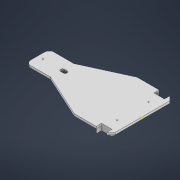
# Autodesk Inventor part: Base
Saved by Autodesk Inventor 2022 (Build 260153000, 153)
## iProperties
Created: 2022-06-09
Part Number: Base
Material: Generic
Document SubType Name: Modeling
Designer: Gugarauj07
Density: 1 g/cm^3
Appearance: Default
Author: Gugarauj07
Autodesk Inventor part; units mm, degrees
ref_plane "YZ Plane" through (0, 0, 0) normal (1, 0, 0) x (0, 1, 0)
ref_plane "XZ Plane" through (0, 0, 0) normal (0, 1, 0) x (-1, 0, 0)
ref_plane "XY Plane" through (0, 0, 0) normal (0, 0, 1) x (1, 0, 0)
sketch "Sketch1" plane through (0, 0, 0) normal (0, 1, 0) x (-1, 0, 0)
  line L0 (0, 0) -> (0, 300)
  line L1 (0, 300) -> (350, 300)
  line L2 (350, 300) -> (1000, 100)
  line L3 (0, 0) -> (1000, 0)
  line L4 (1000, 100) -> (1000, 0)
  line L5 (0, 0) -> (0, -300)
  line L6 (0, -300) -> (350, -300)
  line L7 (350, -300) -> (1000, -100)
  line L8 (1000, -100) -> (1000, 0)
  line L9 (350, 300) -> (350, -300)
  dimension "d12" = 300
  dimension "d13" = 350
  dimension "d16" = 100
  constraints: 20 end point, 3 symmetric about line, 2 vertical, 1 horizontal, 1 perpendicular
  measures "d12" distance of L0.start L0.end
  measures "d13" distance of L0.end L1.end
  measures "d16" distance of L2.end L3.end
extrude "Extrusion1" add sketch "Sketch1" along normal blind 20
fillet "Fillet1" radius 50 1 edges at (-1000, 10, 100)
fillet "Fillet2" radius 50 1 edges at (-1000, 10, -100)
chamfer "Chamfer1" distance 40 angle 45 1 edges at (0, 10, -300)
chamfer "Chamfer2" distance 40 angle 45 1 edges at (0, 10, 300)
sketch "Sketch3" plane through (0, 20, 0) normal (0, 1, 0) x (1, 0, 0)
  point P0 (0, 0)
sketch "Sketch4" plane through (0, 20, 0) normal (0, 1, 0) x (1, 0, 0)
  point P0 (0, 0)
sketch "Sketch5" plane through (0, 20, 0) normal (0, 1, 0) x (1, 0, 0)
  line L0 (-780, 0) -> (-720, 0) construction
  line L1 (-762.5, -17.5) -> (-737.5, -17.5)
  line L2 (-737.5, 17.5) -> (-762.5, 17.5)
  arc A0 (-762.5, 17.5) -> (-762.5, -17.5) centre (-762.5, 0) ccw
  arc A1 (-737.5, -17.5) -> (-737.5, 17.5) centre (-737.5, 0) ccw
  line L3 (-1000, 63.0713) -> (-1000, -63.0713) projected
  point P0 (0, 0)
  point P1 (-750, 0)
  dimension "d27" = 60
  dimension "d28" = 35
  constraints: 8 end point, 6 point on circle, 4 tangent, 2 centre point, 2 point on line, 1 horizontal, 1 midpoint, 1 parallel
  measures "d27" distance of L0.start L0.end
  measures "d28" diameter of A1
extrude "Extrusion2" cut sketch "Sketch5" against normal blind 20
sketch "Sketch6" plane through (0, 20, 0) normal (0, 1, 0) x (1, 0, 0)
  line L0 (-1000, 63.0713) -> (-1000, -63.0713) projected
  line L1 (-1000, 0) -> (-950, 0)
  point P0 (0, 0)
  dimension "d33" = 50
  constraints: 2 end point, 1 horizontal, 1 midpoint
  measures "d33" distance of L1.start L1.end
hole "Hole1" at (-950, 20, 0) direction (0, -1, 0) diameter 10 end through all
sketch "Sketch7" plane through (0, 0, 0) normal (0, -1, 0) x (1, 0, 0)
  line L0 (-350, 300) -> (-40, 300) projected
  line L1 (0, -260) -> (-40, -300) projected
  line L2 (-40, 300) -> (-40, -300)
  line L3 (-40, -300) -> (-140, -300)
  line L4 (-140, -300) -> (-140, 300)
  line L5 (-140, 300) -> (-40, 300)
  point P0 (0, 0)
  dimension "d41" = 100
  constraints: 8 end point, 2 parallel, 1 perpendicular, 1 vertical
  measures "d41" distance of L1.end L3.end
extrude "Extrusion3" add sketch "Sketch7" along normal blind 40
sketch "Sketch8" plane through (0, -40, 0) normal (0, -1, 0) x (1, 0, 0)
  line L0 (-350, 300) -> (-40, 300) projected
  circle A0 centre (-91.5513, 150) radius 5
  line L1 (-40, -300) -> (-40, 300) projected
  line L2 (-40, 0) -> (-140, 0)
  line L3 (-140, -300) -> (-140, 300) projected
  circle A1 centre (-91.5513, -150) radius 5
  point P0 (0, 0)
  dimension "d45" = 10
  constraints: 2 centre point, 2 end point, 2 midpoint, 1 symmetric about line, 1 other
  measures "d45" diameter of A0
extrude "Extrusion4" cut sketch "Sketch8" against normal blind 60 contours A0 | A1
sketch "Sketch9" plane through (0, -40, 0) normal (0, -1, 0) x (1, 0, 0)
  line L0 (-40, -300) -> (-350, -300) projected
  line L1 (-139.5196, -300) -> (-39.5196, -300)
  line L2 (-39.5196, -300) -> (-39.5196, -250)
  line L3 (-39.5196, -250) -> (-139.5196, -250)
  line L4 (-139.5196, -250) -> (-139.5196, -300)
  line L5 (-40, -300) -> (-40, 300) projected
  line L6 (-40, 0) -> (-139.5196, 0)
  line L7 (-40, 300) -> (-350, 300)
  line L8 (-39.5196, 300) -> (-39.5196, 250)
  line L9 (-39.5196, 250) -> (-139.5196, 250)
  line L10 (-139.5196, 250) -> (-139.5196, 300)
  point P0 (0, 0)
  point P1 (-40, 250)
  point P2 (-40, -250)
  dimension "d48" = 100
  dimension "d49" = 50
  constraints: 18 end point, 5 symmetric about line, 2 horizontal, 2 parallel, 2 point on line, 1 midpoint, 1 perpendicular
  measures "d48" distance of L3.end L2.end
  measures "d49" distance of L2.end L1.end
extrude "Extrusion5" cut sketch "Sketch9" against normal blind 60 contours L0 L4 L3 L5 | L9 L10 L7 L5
sketch "Sketch10" plane through (0, 20, 0) normal (0, 1, 0) x (1, 0, 0)
  line L0 (-350, 300) -> (-964.7043, 110.8602) projected
  line L1 (-964.7043, 110.8602) -> (-764.7043, 110.8602)
  line L2 (-764.7043, 110.8602) -> (-350, 300)
  line L3 (-964.7043, -110.8602) -> (-350, -300) projected
  line L4 (-964.7043, -110.8602) -> (-764.7043, -110.8602)
  line L5 (-764.7043, -110.8602) -> (-350, -300)
  point P0 (0, 0)
  dimension "d53" = 200
  constraints: 8 end point, 2 horizontal
  measures "d53" distance of L0.end L1.end
extrude "Extrusion6" cut sketch "Sketch10" against normal blind 20
body "Solid1"
